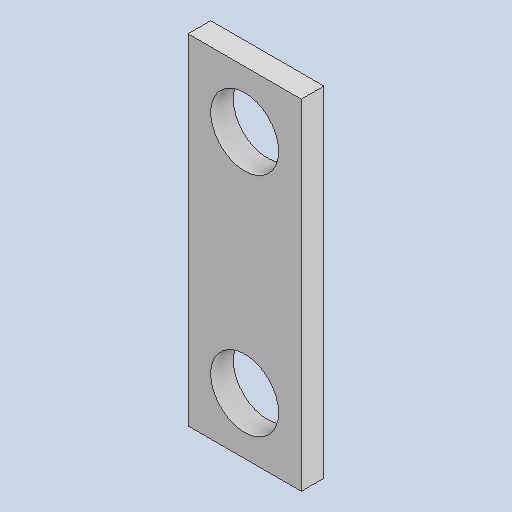
# Autodesk Inventor part: 指先
Saved by Autodesk Inventor 2022 (Build 260153070, 153G)
## iProperties
Created: 2022-10-03
Part Number: 指先
Material: 一般
Document SubType Name: Modeling
Designer: hirok
Density: 1 g/cm^3
Appearance: 既定
Author: hirok
Autodesk Inventor part; units mm, degrees
ref_plane "YZ Plane" through (0, 0, 0) normal (1, 0, 0) x (0, 1, 0)
ref_plane "XZ Plane" through (0, 0, 0) normal (0, 1, 0) x (-1, 0, 0)
ref_plane "XY Plane" through (0, 0, 0) normal (0, 0, 1) x (1, 0, 0)
sketch "スケッチ1" plane through (0, 0, 0) normal (0, 0, 1) x (1, 0, 0)
  line L0 (0, 0) -> (10, 0)
  line L1 (10, 0) -> (10, 30)
  line L2 (10, 30) -> (0, 30)
  line L3 (0, 30) -> (0, 0)
  dimension "d0" = 10
  dimension "d1" = 30
  constraints: 8 end point, 2 parallel, 1 horizontal, 1 perpendicular
  measures "d0" distance of L0.start L0.end
  measures "d1" distance of L0.end L1.end
extrude "押し出し1" add sketch "スケッチ1" along normal blind 2
sketch "スケッチ2" plane through (0, 0, 2) normal (0, 0, 1) x (1, 0, 0)
  line L0 (0, 0) -> (10, 0) projected
  line L1 (10, 30) -> (0, 30) projected
  line L2 (0, 30) -> (0, 0) projected
  point P0 (5, 5)
  point P1 (5, 25)
  dimension "d4" = 5
  dimension "d12" = 5
  dimension "d13" = 5
  measures "d4" distance from line of L0 point (5, 5)
  measures "d12" distance from line of point (5, 25) L1
  measures "d13" distance from line of L2 point (5, 5)
hole "穴1" at (5, 5, 2) at (5, 25, 2) direction (0, 0, -1) diameter 6 end through all
